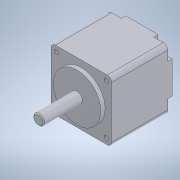
# Autodesk Inventor part: NEMA 11
Saved by Autodesk Inventor 2022 (Build 260153000, 153)
## iProperties
Created: 2022-03-30
Part Number: NEMA 11
Material: Generic
Document SubType Name: Modeling
Designer: Nick
Density: 1 g/cm^3
Appearance: Default
Mass: 0.60083 g
Surface Area: 5.70199 cm^2
Volume: 0.60083 cm^3
Sending System: SolidWorks 2021
Preprocessor: SwSTEP 2.0
MotorHeightBase: 28.000 mm
Title: NEMA 11
Autodesk Inventor part; units mm, degrees
ref_plane "YZ Plane" through (0, 0, 0) normal (1, 0, 0) x (0, 1, 0)
ref_plane "XZ Plane" through (0, 0, 0) normal (0, 1, 0) x (-1, 0, 0)
ref_plane "XY Plane" through (0, 0, 0) normal (0, 0, 1) x (1, 0, 0)
sketch "Sketch6" plane through (0, 0, 0) normal (0, 0, 1) x (1, 0, 0)
  line L0 (20.7414, 11.7807) -> (48.7414, 11.7807)
  line L1 (48.7414, 11.7807) -> (48.7414, -16.2193)
  line L2 (48.7414, -16.2193) -> (20.7414, -16.2193)
  line L3 (20.7414, -16.2193) -> (20.7414, 11.7807)
  point P0 (0, 0)
  dimension "d10" = 28
  constraints: 8 end point, 2 parallel, 2 perpendicular, 1 horizontal
  measures "d10" distance of L0.start L0.end
extrude "Extrusion6" add sketch "Sketch6" against normal blind 28
sketch "Sketch7" plane through (0, 0, 0) normal (0, 0, 1) x (1, 0, 0)
  line L0 (48.7414, 11.7807) -> (20.7414, 11.7807) projected
  line L1 (20.7414, 11.7807) -> (20.7414, -16.2193) projected
  line L2 (48.7414, -16.2193) -> (48.7414, 11.7807) projected
  line L3 (20.7414, -16.2193) -> (48.7414, -16.2193) projected
  point P0 (0, 0)
  point P1 (23.2414, 9.2807)
  point P2 (46.2414, 9.2807)
  point P3 (46.2414, -13.7193)
  point P4 (23.2414, -13.7193)
  point P5 (46.7414, 11.7807)
  point P6 (22.7414, 11.7807)
  point P7 (20.7414, 9.7807)
  point P8 (20.7414, -14.2193)
  point P9 (48.7414, -14.2193)
  point P10 (48.7414, 9.7807)
  point P11 (22.7414, -16.2193)
  point P12 (46.7414, -16.2193)
  dimension "d14" = 2.5
  dimension "d15" = 2.5
  dimension "d16" = 2.5
  dimension "d17" = 2.5
  constraints: 2 horizontal alignment, 2 vertical alignment
  measures "d14" distance from line of L0 point (23.241, 9.281)
  measures "d15" distance from line of L1 point (23.241, 9.281)
  measures "d16" distance from line of L2 point (46.241, -13.719)
  measures "d17" distance from line of L3 point (46.241, -13.719)
hole "Hole1" at (23.2414, 9.2807, 0) at (46.2414, 9.2807, 0) at (46.2414, -13.7193, 0) at (23.2414, -13.7193, 0) direction (0, 0, -1) diameter 2.013 depth 4.5 thread size "M2.5x0.45" class "6H" standard "ANSI Metric M Profile"
sketch "Sketch8" plane through (0, 0, 0) normal (0, 0, 1) x (1, 0, 0)
  circle A0 centre (34.7414, -2.2193) radius 11
  line L0 (48.7414, -16.2193) -> (48.7414, 11.7807) projected
  line L1 (48.7414, 11.7807) -> (20.7414, 11.7807) projected
  point P0 (0, 0)
  point P1 (48.7414, -2.2193)
  point P2 (48.7414, -14.2193)
  point P3 (48.7414, 9.7807)
  point P4 (34.7414, 11.7807)
  point P5 (46.7414, 11.7807)
  point P6 (22.7414, 11.7807)
  dimension "d25" = 22
  constraints: 2 midpoint, 1 centre point, 1 horizontal alignment, 1 vertical alignment
  measures "d25" diameter of A0
extrude "Extrusion7" add sketch "Sketch8" along normal blind 2
sketch "Sketch9" plane through (34.7414, -2.2193, 2) normal (0, 0, 1) x (1, 0, 0)
  circle A0 centre (0, 0) radius 2.5
  circle A1 centre (0, 0) radius 11 projected
  point P0 (-34.7414, 2.2193)
  dimension "d28" = 5
  constraints: 1 centre point, 1 coincident
  measures "d28" diameter of A0
extrude "Extrusion8" add sketch "Sketch9" along normal blind 18 contours A0
chamfer "Chamfer1" distance 0.5 angle 45 1 edges at (32.2414, -2.2193, 20)
sketch "Sketch10" plane through (0, 0, -28) normal (0, 0, -1) x (-1, 0, 0)
  line L0 (-20.7414, 11.7807) -> (-27.2414, 11.7807)
  line L1 (-27.2414, 11.7807) -> (-27.2414, 5.2807)
  line L2 (-27.2414, 5.2807) -> (-20.7414, 5.2807)
  line L3 (-20.7414, 5.2807) -> (-20.7414, 11.7807)
  line L4 (-20.7414, -16.2193) -> (-27.2414, -16.2193)
  line L5 (-27.2414, -16.2193) -> (-27.2414, -9.7193)
  line L6 (-27.2414, -9.7193) -> (-20.7414, -9.7193)
  line L7 (-20.7414, -9.7193) -> (-20.7414, -16.2193)
  line L8 (-48.7414, -16.2193) -> (-42.2414, -16.2193)
  line L9 (-42.2414, -16.2193) -> (-42.2414, -9.7193)
  line L10 (-42.2414, -9.7193) -> (-48.7414, -9.7193)
  line L11 (-48.7414, -9.7193) -> (-48.7414, -16.2193)
  line L12 (-42.2414, 11.7807) -> (-48.7414, 11.7807)
  line L13 (-48.7414, 11.7807) -> (-48.7414, 5.2807)
  line L14 (-48.7414, 5.2807) -> (-42.2414, 5.2807)
  line L15 (-42.2414, 5.2807) -> (-42.2414, 11.7807)
  line L16 (-20.7414, -16.2193) -> (-20.7414, 11.7807) projected
  line L17 (-20.7414, 11.7807) -> (-48.7414, 11.7807) projected
  line L18 (-48.7414, -16.2193) -> (-20.7414, -16.2193) projected
  line L19 (-48.7414, 11.7807) -> (-48.7414, -16.2193) projected
  point P0 (0, 0)
  point P1 (-20.7414, -14.2193)
  point P2 (-20.7414, 9.7807)
  point P3 (-22.7414, 11.7807)
  point P4 (-46.7414, 11.7807)
  point P5 (-46.7414, -16.2193)
  point P6 (-22.7414, -16.2193)
  point P7 (-48.7414, 9.7807)
  point P8 (-48.7414, -14.2193)
  dimension "d34" = 6.5
  constraints: 32 end point, 8 parallel, 7 equal length, 6 collinear, 4 horizontal, 4 perpendicular, 2 point on line
  measures "d34" distance between parallel lines of L2 L0
extrude "Extrusion9" cut sketch "Sketch10" against normal blind 2 contours L3 L2 L1 L0 | L15 L14 L13 L12 | L7 L4 L5 L6 | L10 L9 L8 L11
sketch "Sketch11" plane through (0, 0, -26) normal (0, 0, -1) x (-1, 0, 0)
  circle A0 centre (-23.2414, -13.7193) radius 1.0065 projected
  circle A1 centre (-23.2414, 9.2807) radius 1.0065 projected
  circle A2 centre (-46.2414, -13.7193) radius 1.0065 projected
  circle A3 centre (-46.2414, 9.2807) radius 1.0065 projected
  point P0 (0, 0)
extrude "Extrusion10" cut sketch "Sketch11" against normal blind 4.5
fillet "Fillet2" radius 2 8 edges at (20.7414, 11.7807, -13) (48.7414, 11.7807, -13) (20.7414, -16.2193, -13) (48.7414, -16.2193, -13) (27.2414, -9.7193, -27) (27.2414, 5.2807, -27) (42.2414, 5.2807, -27) (42.2414, -9.7193, -27)
equation "\"d11\" = MotorHeightBase"
equation "\"d17\" = d15"
equation "\"MotorHeightBase\" = 28"
body "Solid4"
